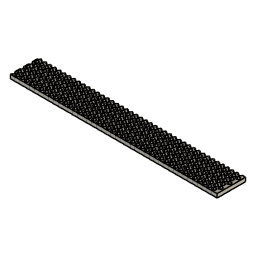
newmeshhoneycomb (Autodesk Fusion 360 design; units mm, degrees)
Autodesk Fusion 360 part; units mm, degrees
(part 1 of 3)
sketch "Sketch1" plane through (0, 0, 0) normal (0, 0, 1) x (1, 0, 0)
  line L0 (-30.9287, -0.75) -> (-29.6296, -1.5)
  line L1 (-30.9287, 0.75) -> (-30.9287, -0.75)
  line L2 (-29.6296, 1.5) -> (-30.9287, 0.75)
  line L3 (-33.3333, -1.5) -> (-32.0343, -0.75)
  line L4 (-34.6324, -0.75) -> (-33.3333, -1.5)
  line L5 (-34.6324, 0.75) -> (-34.6324, -0.75)
  line L6 (-33.3333, 1.5) -> (-34.6324, 0.75)
  line L7 (-32.0343, 0.75) -> (-33.3333, 1.5)
  line L8 (-32.0343, -0.75) -> (-32.0343, 0.75)
  line L9 (-29.225, -2.7141) -> (-29.225, -4.2141)
  line L10 (-30.3306, -2.7141) -> (-31.6296, -1.9641)
  line L11 (-31.6296, -1.9641) -> (-32.9287, -2.7141)
  line L12 (-32.9287, -2.7141) -> (-32.9287, -4.2141)
  line L13 (-32.9287, -4.2141) -> (-31.6296, -4.9641)
  line L14 (-31.6296, -4.9641) -> (-30.3306, -4.2141)
  line L15 (-30.3306, -4.2141) -> (-30.3306, -2.7141)
  line L16 (-34.0343, -2.7141) -> (-35.3333, -1.9641)
  line L17 (-35.3333, -1.9641) -> (-36.6324, -2.7141)
  line L18 (-36.6324, -2.7141) -> (-36.6324, -4.2141)
  line L19 (-36.6324, -4.2141) -> (-35.3333, -4.9641)
  line L20 (-35.3333, -4.9641) -> (-34.0343, -4.2141)
  line L21 (-34.0343, -4.2141) -> (-34.0343, -2.7141)
  line L22 (-31.0583, -5.8895) -> (-31.0583, -7.3895)
  line L23 (-39.1667, -8.6036) -> (-40.4657, -9.3536)
  line L24 (-34.762, -5.8895) -> (-34.762, -7.3895)
  line L25 (-40.4657, -9.3536) -> (-40.4657, -10.8536)
  line L26 (-29.3546, -9.3536) -> (-29.3546, -10.8536)
  line L27 (-33.463, -5.1395) -> (-34.762, -5.8895)
  line L28 (-31.0583, -7.3895) -> (-29.7593, -8.1395)
  line L29 (-30.4602, -10.8536) -> (-30.4602, -9.3536)
  line L30 (-37.8676, -10.8536) -> (-37.8676, -9.3536)
  line L31 (-32.1639, -7.3895) -> (-32.1639, -5.8895)
  line L32 (-39.1667, -11.6036) -> (-37.8676, -10.8536)
  line L33 (-36.762, -10.8536) -> (-35.463, -11.6036)
  line L34 (-35.8676, -7.3895) -> (-35.8676, -5.8895)
  line L35 (-33.0583, -10.8536) -> (-31.7593, -11.6036)
  line L36 (-35.463, -11.6036) -> (-34.1639, -10.8536)
  line L37 (-29.7593, -5.1395) -> (-31.0583, -5.8895)
  line L38 (-33.0583, -9.3536) -> (-33.0583, -10.8536)
  line L39 (-30.4602, -9.3536) -> (-31.7593, -8.6036)
  line L40 (-31.7593, -11.6036) -> (-30.4602, -10.8536)
  line L41 (-34.1639, -9.3536) -> (-35.463, -8.6036)
  line L42 (-32.1639, -5.8895) -> (-33.463, -5.1395)
  line L43 (-35.463, -8.6036) -> (-36.762, -9.3536)
  line L44 (-36.762, -9.3536) -> (-36.762, -10.8536)
  line L45 (-34.762, -7.3895) -> (-33.463, -8.1395)
  line L46 (-34.1639, -10.8536) -> (-34.1639, -9.3536)
  line L47 (-38.4657, -5.8895) -> (-38.4657, -7.3895)
  line L48 (-33.463, -8.1395) -> (-32.1639, -7.3895)
  line L49 (-31.7593, -8.6036) -> (-33.0583, -9.3536)
  line L50 (-37.8676, -9.3536) -> (-39.1667, -8.6036)
  line L51 (-35.8676, -5.8895) -> (-37.1667, -5.1395)
  line L52 (-37.1667, -8.1395) -> (-35.8676, -7.3895)
  line L53 (-37.1667, -5.1395) -> (-38.4657, -5.8895)
  line L54 (-38.4657, -7.3895) -> (-37.1667, -8.1395)
  line L55 (-40.4657, -10.8536) -> (-39.1667, -11.6036)
  line L56 (-34.8916, -12.5291) -> (-34.8916, -14.0291)
  line L57 (-43, -15.2432) -> (-44.299, -15.9932)
  line L58 (-38.5953, -12.5291) -> (-38.5953, -14.0291)
  line L59 (-44.299, -15.9932) -> (-44.299, -17.4932)
  line L60 (-33.1879, -15.9932) -> (-33.1879, -17.4932)
  line L61 (-37.2963, -11.7791) -> (-38.5953, -12.5291)
  line L62 (-34.8916, -14.0291) -> (-33.5926, -14.7791)
  line L63 (-34.2936, -17.4932) -> (-34.2936, -15.9932)
  line L64 (-33.1879, -17.4932) -> (-31.8889, -18.2432)
  line L65 (-33.5926, -14.7791) -> (-32.2936, -14.0291)
  line L66 (-30.5899, -15.9932) -> (-31.8889, -15.2432)
  line L67 (-30.5899, -17.4932) -> (-30.5899, -15.9932)
  line L68 (-29.8889, -11.7791) -> (-31.1879, -12.5291)
  line L69 (-29.4842, -15.9932) -> (-29.4842, -17.4932)
  line L70 (-31.8889, -18.2432) -> (-30.5899, -17.4932)
  line L71 (-41.701, -17.4932) -> (-41.701, -15.9932)
  line L72 (-35.9973, -14.0291) -> (-35.9973, -12.5291)
  line L73 (-43, -18.2432) -> (-41.701, -17.4932)
  line L74 (-31.8889, -15.2432) -> (-33.1879, -15.9932)
  line L75 (-40.5953, -17.4932) -> (-39.2963, -18.2432)
  line L76 (-39.701, -14.0291) -> (-39.701, -12.5291)
  line L77 (-36.8916, -17.4932) -> (-35.5926, -18.2432)
  line L78 (-39.2963, -18.2432) -> (-37.9973, -17.4932)
  line L79 (-31.1879, -14.0291) -> (-29.8889, -14.7791)
  line L80 (-33.5926, -11.7791) -> (-34.8916, -12.5291)
  line L81 (-36.8916, -15.9932) -> (-36.8916, -17.4932)
  line L82 (-34.2936, -15.9932) -> (-35.5926, -15.2432)
  line L83 (-35.5926, -18.2432) -> (-34.2936, -17.4932)
  line L84 (-37.9973, -15.9932) -> (-39.2963, -15.2432)
  line L85 (-32.2936, -12.5291) -> (-33.5926, -11.7791)
  line L86 (-35.9973, -12.5291) -> (-37.2963, -11.7791)
  line L87 (-39.2963, -15.2432) -> (-40.5953, -15.9932)
  line L88 (-40.5953, -15.9932) -> (-40.5953, -17.4932)
  line L89 (-31.1879, -12.5291) -> (-31.1879, -14.0291)
  line L90 (-38.5953, -14.0291) -> (-37.2963, -14.7791)
  line L91 (-37.9973, -17.4932) -> (-37.9973, -15.9932)
  line L92 (-32.2936, -14.0291) -> (-32.2936, -12.5291)
  line L93 (-42.299, -12.5291) -> (-42.299, -14.0291)
  line L94 (-37.2963, -14.7791) -> (-35.9973, -14.0291)
  line L95 (-35.5926, -15.2432) -> (-36.8916, -15.9932)
  line L96 (-41.701, -15.9932) -> (-43, -15.2432)
  line L97 (-39.701, -12.5291) -> (-41, -11.7791)
  line L98 (-41, -14.7791) -> (-39.701, -14.0291)
  line L99 (-41, -11.7791) -> (-42.299, -12.5291)
  line L100 (-42.299, -14.0291) -> (-41, -14.7791)
  line L101 (-44.299, -17.4932) -> (-43, -18.2432)
  line L102 (-38.725, -19.1686) -> (-38.725, -20.6686)
  line L103 (-42.4287, -19.1686) -> (-42.4287, -20.6686)
  line L104 (-41.1296, -18.4186) -> (-42.4287, -19.1686)
  line L105 (-38.725, -20.6686) -> (-37.4259, -21.4186)
  line L106 (-37.4259, -21.4186) -> (-36.1269, -20.6686)
  line L107 (-33.7222, -18.4186) -> (-35.0213, -19.1686)
  line L108 (-31.3176, -20.6686) -> (-30.0185, -21.4186)
  line L109 (-33.7222, -21.4186) -> (-32.4232, -20.6686)
  line L110 (-39.8306, -20.6686) -> (-39.8306, -19.1686)
  line L111 (-32.4232, -20.6686) -> (-32.4232, -19.1686)
  line L112 (-32.4232, -19.1686) -> (-33.7222, -18.4186)
  line L113 (-43.5343, -20.6686) -> (-43.5343, -19.1686)
  line L114 (-35.0213, -20.6686) -> (-33.7222, -21.4186)
  line L115 (-37.4259, -18.4186) -> (-38.725, -19.1686)
  line L116 (-30.0185, -18.4186) -> (-31.3176, -19.1686)
  line L117 (-36.1269, -19.1686) -> (-37.4259, -18.4186)
  line L118 (-39.8306, -19.1686) -> (-41.1296, -18.4186)
  line L119 (-31.3176, -19.1686) -> (-31.3176, -20.6686)
  line L120 (-35.0213, -19.1686) -> (-35.0213, -20.6686)
  line L121 (-42.4287, -20.6686) -> (-41.1296, -21.4186)
  line L122 (-36.1269, -20.6686) -> (-36.1269, -19.1686)
  line L123 (-46.1324, -19.1686) -> (-46.1324, -20.6686)
  line L124 (-41.1296, -21.4186) -> (-39.8306, -20.6686)
  line L125 (-43.5343, -19.1686) -> (-44.8333, -18.4186)
  line L126 (-44.8333, -21.4186) -> (-43.5343, -20.6686)
  line L127 (-44.8333, -18.4186) -> (-46.1324, -19.1686)
  line L128 (-46.1324, -20.6686) -> (-44.8333, -21.4186)
  line L129 (-101.9101, -19.1686) -> (-101.9101, -20.6686)
  line L130 (-99.3121, -19.1686) -> (-100.6111, -18.4186)
  line L131 (-95.5343, -19.1686) -> (-96.8333, -18.4186)
  line L132 (-98.1324, -19.1686) -> (-98.1324, -20.6686)
  line L133 (-95.5343, -20.6686) -> (-95.5343, -19.1686)
  line L134 (-96.8333, -18.4186) -> (-98.1324, -19.1686)
  line L135 (-100.6111, -21.4186) -> (-99.3121, -20.6686)
  line L136 (-103.0158, -19.1686) -> (-104.3148, -18.4186)
  line L137 (-106.7195, -19.1686) -> (-108.0185, -18.4186)
  line L138 (-109.3176, -20.6686) -> (-108.0185, -21.4186)
  line L139 (-110.4232, -19.1686) -> (-111.7222, -18.4186)
  line L140 (-103.7805, -15.9932) -> (-103.7805, -17.4932)
  line L141 (-102.8861, -12.5291) -> (-104.1852, -11.7791)
  line L142 (-106.5899, -14.0291) -> (-106.5899, -12.5291)
  line L143 (-108.5899, -15.9932) -> (-109.8889, -15.2432)
  line L144 (-105.4842, -14.0291) -> (-104.1852, -14.7791)
  line L145 (-106.1852, -15.2432) -> (-107.4842, -15.9932)
  line L146 (-109.1879, -12.5291) -> (-109.1879, -14.0291)
  line L147 (-105.4842, -12.5291) -> (-105.4842, -14.0291)
  line L148 (-107.4842, -17.4932) -> (-106.1852, -18.2432)
  line L149 (-107.8889, -11.7791) -> (-109.1879, -12.5291)
  line L150 (-109.8889, -15.2432) -> (-111.1879, -15.9932)
  line L151 (-88.1269, -20.6686) -> (-88.1269, -19.1686)
  line L152 (-91.8306, -19.1686) -> (-93.1296, -18.4186)
  line L153 (-93.1296, -21.4186) -> (-91.8306, -20.6686)
  line L154 (-90.725, -20.6686) -> (-89.4259, -21.4186)
  line L155 (-94.4287, -19.1686) -> (-94.4287, -20.6686)
  line L156 (-94.4287, -20.6686) -> (-93.1296, -21.4186)
  line L157 (-89.4259, -21.4186) -> (-88.1269, -20.6686)
  line L158 (-90.725, -19.1686) -> (-90.725, -20.6686)
  line L159 (-93.1296, -18.4186) -> (-94.4287, -19.1686)
  line L160 (-89.4259, -18.4186) -> (-90.725, -19.1686)
  line L161 (-101.9101, -20.6686) -> (-100.6111, -21.4186)
  line L162 (-96.8333, -21.4186) -> (-95.5343, -20.6686)
  line L163 (-99.3121, -20.6686) -> (-99.3121, -19.1686)
  line L164 (-95.4787, -14.0291) -> (-95.4787, -12.5291)
  line L165 (-96.7778, -11.7791) -> (-98.0768, -12.5291)
  line L166 (-97.4787, -15.9932) -> (-98.7778, -15.2432)
  line L167 (-101.1824, -15.9932) -> (-102.4815, -15.2432)
  line L168 (-98.7778, -15.2432) -> (-100.0768, -15.9932)
  line L169 (-96.7778, -14.7791) -> (-95.4787, -14.0291)
  line L170 (-101.1824, -17.4932) -> (-101.1824, -15.9932)
  line L171 (-95.4787, -12.5291) -> (-96.7778, -11.7791)
  line L172 (-101.7805, -12.5291) -> (-101.7805, -14.0291)
  line L173 (-98.7778, -18.2432) -> (-97.4787, -17.4932)
  line L174 (-111.3333, 1.5) -> (-112.6324, 0.75)
  line L175 (-99.1824, -12.5291) -> (-100.4815, -11.7791)
  line L176 (-100.4815, -14.7791) -> (-99.1824, -14.0291)
  line L177 (-111.463, -8.1395) -> (-110.1639, -7.3895)
  line L178 (-98.0768, -12.5291) -> (-98.0768, -14.0291)
  line L179 (-104.1852, -14.7791) -> (-102.8861, -14.0291)
  line L180 (-107.4842, -15.9932) -> (-107.4842, -17.4932)
  line L181 (-104.8861, -17.4932) -> (-104.8861, -15.9932)
  line L182 (-106.1852, -18.2432) -> (-104.8861, -17.4932)
  line L183 (-104.1852, -11.7791) -> (-105.4842, -12.5291)
  line L184 (-111.1879, -15.9932) -> (-111.1879, -17.4932)
  line L185 (-111.1879, -17.4932) -> (-109.8889, -18.2432)
  line L186 (-100.6111, -18.4186) -> (-101.9101, -19.1686)
  line L187 (-98.1324, -20.6686) -> (-96.8333, -21.4186)
  line L188 (-90.5953, -12.5291) -> (-90.5953, -14.0291)
  line L189 (-91.701, -14.0291) -> (-91.701, -12.5291)
  line L190 (-88.8916, -15.9932) -> (-88.8916, -17.4932)
  line L191 (-91.2963, -18.2432) -> (-89.9973, -17.4932)
  line L192 (-93, -11.7791) -> (-94.299, -12.5291)
  line L193 (-89.9973, -15.9932) -> (-91.2963, -15.2432)
  line L194 (-91.701, -12.5291) -> (-93, -11.7791)
  line L195 (-92.5953, -15.9932) -> (-92.5953, -17.4932)
  line L196 (-91.2963, -15.2432) -> (-92.5953, -15.9932)
  line L197 (-94.299, -12.5291) -> (-94.299, -14.0291)
  line L198 (-111.5926, -14.7791) -> (-110.2936, -14.0291)
  line L199 (-89.2963, -11.7791) -> (-90.5953, -12.5291)
  line L200 (-92.5953, -17.4932) -> (-91.2963, -18.2432)
  line L201 (-95, -18.2432) -> (-93.701, -17.4932)
  line L202 (-93.701, -17.4932) -> (-93.701, -15.9932)
  line L203 (-112.6324, -0.75) -> (-111.3333, -1.5)
  line L204 (-111.7222, -21.4186) -> (-110.4232, -20.6686)
  line L205 (-103.0158, -20.6686) -> (-103.0158, -19.1686)
  line L206 (-104.3148, -18.4186) -> (-105.6139, -19.1686)
  line L207 (-105.6139, -20.6686) -> (-104.3148, -21.4186)
  line L208 (-109.3176, -19.1686) -> (-109.3176, -20.6686)
  line L209 (-91.8306, -20.6686) -> (-91.8306, -19.1686)
  line L210 (-88.1269, -19.1686) -> (-89.4259, -18.4186)
  line L211 (-94.299, -14.0291) -> (-93, -14.7791)
  line L212 (-89.9973, -17.4932) -> (-89.9973, -15.9932)
  line L213 (-87.9973, -12.5291) -> (-89.2963, -11.7791)
  line L214 (-93, -14.7791) -> (-91.701, -14.0291)
  line L215 (-58.1639, -7.3895) -> (-58.1639, -5.8895)
  line L216 (-89.8121, -4.2141) -> (-89.8121, -2.7141)
  line L217 (-66.4657, -9.3536) -> (-66.4657, -10.8536)
  line L218 (-57.6296, -1.9641) -> (-58.9287, -2.7141)
  line L219 (-63.1111, -1.5) -> (-61.8121, -0.75)
  line L220 (-93.5158, -2.7141) -> (-94.8148, -1.9641)
  line L221 (-71.2195, -4.2141) -> (-71.2195, -2.7141)
  line L222 (-73.0528, -5.8895) -> (-74.3519, -5.1395)
  line L223 (-103.9259, -1.5) -> (-102.6269, -0.75)
  line L224 (-52.0556, -8.1395) -> (-50.7565, -7.3895)
  line L225 (-63.8121, -4.2141) -> (-63.8121, -2.7141)
  line L226 (-56.9287, -0.75) -> (-55.6296, -1.5)
  line L227 (-91.1111, -1.9641) -> (-92.4101, -2.7141)
  line L228 (-45.3491, -10.8536) -> (-45.3491, -9.3536)
  line L229 (-58.9287, -4.2141) -> (-57.6296, -4.9641)
  line L230 (-105.225, -0.75) -> (-103.9259, -1.5)
  line L231 (-73.8176, -4.2141) -> (-72.5185, -4.9641)
  line L232 (-90.4657, -5.8895) -> (-90.4657, -7.3895)
  line L233 (-68.8148, -4.9641) -> (-67.5158, -4.2141)
  line L234 (-75.6509, -7.3895) -> (-74.3519, -8.1395)
  line L235 (-52.0556, -5.1395) -> (-53.3546, -5.8895)
  line L236 (-92.8148, -1.5) -> (-91.5158, -0.75)
  line L237 (-42.8148, -1.9641) -> (-44.1139, -2.7141)
  line L238 (-92.4657, -9.3536) -> (-92.4657, -10.8536)
  line L239 (-74.9232, -4.2141) -> (-74.9232, -2.7141)
  line L240 (-63.8676, -9.3536) -> (-65.1667, -8.6036)
  line L241 (-71.2195, -2.7141) -> (-72.5185, -1.9641)
  line L242 (-73.9472, -9.3536) -> (-73.9472, -10.8536)
  line L243 (-53.9259, -1.9641) -> (-55.225, -2.7141)
  line L244 (-54.4602, -5.8895) -> (-55.7593, -5.1395)
  line L245 (-94.2435, -7.3895) -> (-92.9444, -8.1395)
  line L246 (-74.3519, -8.1395) -> (-73.0528, -7.3895)
  line L247 (-70.1139, -2.7141) -> (-70.1139, -4.2141)
  line L248 (-44.2435, -9.3536) -> (-44.2435, -10.8536)
  line L249 (-75.5213, -0.75) -> (-74.2222, -1.5)
  line L250 (-90.4101, -0.75) -> (-89.1111, -1.5)
  line L251 (-103.5213, -4.2141) -> (-102.2222, -4.9641)
  line L252 (-76.2222, -4.9641) -> (-74.9232, -4.2141)
  line L253 (-68.9444, -8.6036) -> (-70.2435, -9.3536)
  line L254 (-104.6269, -4.2141) -> (-104.6269, -2.7141)
  line L255 (-103.5213, -2.7141) -> (-103.5213, -4.2141)
  line L256 (-71.3491, -9.3536) -> (-72.6481, -8.6036)
  line L257 (-74.3519, -5.1395) -> (-75.6509, -5.8895)
  line L258 (-59.3333, -1.5) -> (-58.0343, -0.75)
  line L259 (-93.5158, -4.2141) -> (-93.5158, -2.7141)
  line L260 (-77.5213, -4.2141) -> (-76.2222, -4.9641)
  line L261 (-41.6454, -9.3536) -> (-42.9444, -8.6036)
  line L262 (-65.1111, -4.9641) -> (-63.8121, -4.2141)
  line L263 (-89.8676, -10.8536) -> (-89.8676, -9.3536)
  line L264 (-55.225, -4.2141) -> (-53.9259, -4.9641)
  line L265 (-56.4602, -10.8536) -> (-56.4602, -9.3536)
  line L266 (-74.2222, -1.5) -> (-72.9232, -0.75)
  line L267 (-41.5158, -2.7141) -> (-42.8148, -1.9641)
  line L268 (-73.8176, -2.7141) -> (-73.8176, -4.2141)
  line L269 (-76.2222, -1.9641) -> (-77.5213, -2.7141)
  line L270 (-63.8121, -2.7141) -> (-65.1111, -1.9641)
  line L271 (-47.9472, -9.3536) -> (-47.9472, -10.8536)
  line L272 (-91.1111, -4.9641) -> (-89.8121, -4.2141)
  line L273 (-65.1111, -1.9641) -> (-66.4101, -2.7141)
  line L274 (-54.0556, -8.6036) -> (-55.3546, -9.3536)
  line L275 (-73.0528, -7.3895) -> (-73.0528, -5.8895)
  line L276 (-50.7565, -7.3895) -> (-50.7565, -5.8895)
  line L277 (-94.1139, -0.75) -> (-92.8148, -1.5)
  line L278 (-70.6481, -8.1395) -> (-69.3491, -7.3895)
  line L279 (-49.9101, -20.6686) -> (-48.6111, -21.4186)
  line L280 (-82.9287, -0.75) -> (-81.6296, -1.5)
  line L281 (-78.3148, -21.4186) -> (-77.0158, -20.6686)
  line L282 (-63.9973, -15.9932) -> (-65.2963, -15.2432)
  line L283 (-88.8916, -17.4932) -> (-87.5926, -18.2432)
  line L284 (-49.7805, -14.0291) -> (-48.4815, -14.7791)
  line L285 (-83.8889, -15.2432) -> (-85.1879, -15.9932)
  line L286 (-45.4787, -17.4932) -> (-45.4787, -15.9932)
  line L287 (-60.762, -7.3895) -> (-59.463, -8.1395)
  line L288 (-110.1639, -7.3895) -> (-110.1639, -5.8895)
  line L289 (-83.6296, -4.9641) -> (-82.3306, -4.2141)
  line L290 (-51.0158, -19.1686) -> (-52.3148, -18.4186)
  line L291 (-109.7593, -8.6036) -> (-111.0583, -9.3536)
  line L292 (-48.6111, -18.4186) -> (-49.9101, -19.1686)
  line L293 (-107.3546, -9.3536) -> (-107.3546, -10.8536)
  line L294 (-109.0583, -5.8895) -> (-109.0583, -7.3895)
  line L295 (-78.8861, -17.4932) -> (-78.8861, -15.9932)
  line L296 (-70.299, -17.4932) -> (-69, -18.2432)
  line L297 (-50.4815, -15.2432) -> (-51.7805, -15.9932)
  line L298 (-82.3306, -2.7141) -> (-83.6296, -1.9641)
  line L299 (-61.9973, -12.5291) -> (-63.2963, -11.7791)
  line L300 (-81.7593, -5.1395) -> (-83.0583, -5.8895)
  line L301 (-60.2936, -17.4932) -> (-60.2936, -15.9932)
  line L302 (-101.5213, -0.75) -> (-100.2222, -1.5)
  line L303 (-60.6324, -0.75) -> (-59.3333, -1.5)
  line L304 (-107.7593, -8.1395) -> (-106.4602, -7.3895)
  line L305 (-53.6139, -19.1686) -> (-53.6139, -20.6686)
  line L306 (-50.4815, -18.2432) -> (-49.1824, -17.4932)
  line L307 (-78.1852, -14.7791) -> (-76.8861, -14.0291)
  line L308 (-82.4602, -10.8536) -> (-82.4602, -9.3536)
  line L309 (-85.0583, -9.3536) -> (-85.0583, -10.8536)
  line L310 (-108.4602, -9.3536) -> (-109.7593, -8.6036)
  line L311 (-77.7805, -17.4932) -> (-76.4815, -18.2432)
  line L312 (-79.6139, -20.6686) -> (-78.3148, -21.4186)
  line L313 (-61.0213, -20.6686) -> (-59.7222, -21.4186)
  line L314 (-108.4602, -10.8536) -> (-108.4602, -9.3536)
  line L315 (-46.0768, -12.5291) -> (-46.0768, -14.0291)
  line L316 (-84.2936, -12.5291) -> (-85.5926, -11.7791)
  line L317 (-64.725, -19.1686) -> (-64.725, -20.6686)
  line L318 (-69.5343, -20.6686) -> (-69.5343, -19.1686)
  line L319 (-52.3148, -18.4186) -> (-53.6139, -19.1686)
  line L320 (-111.0583, -9.3536) -> (-111.0583, -10.8536)
  line L321 (-83.0583, -7.3895) -> (-81.7593, -8.1395)
  line L322 (-76.8861, -12.5291) -> (-78.1852, -11.7791)
  line L323 (-52.1852, -11.7791) -> (-53.4842, -12.5291)
  line L324 (-49.9101, -19.1686) -> (-49.9101, -20.6686)
  line L325 (-48.4815, -11.7791) -> (-49.7805, -12.5291)
  line L326 (-76.4815, -18.2432) -> (-75.1824, -17.4932)
  line L327 (-84.9287, -2.7141) -> (-84.9287, -4.2141)
  line L328 (-59.7222, -18.4186) -> (-61.0213, -19.1686)
  line L329 (-109.0583, -7.3895) -> (-107.7593, -8.1395)
  line L330 (-86.6324, -0.75) -> (-85.3333, -1.5)
  line L331 (-50.8861, -14.0291) -> (-50.8861, -12.5291)
  line L332 (-106.4602, -7.3895) -> (-106.4602, -5.8895)
  line L333 (-71.4787, -17.4932) -> (-71.4787, -15.9932)
  line L334 (-72.0768, -14.0291) -> (-70.7778, -14.7791)
  line L335 (-76.8861, -14.0291) -> (-76.8861, -12.5291)
  line L336 (-64.725, -20.6686) -> (-63.4259, -21.4186)
  line L337 (-86.2936, -17.4932) -> (-86.2936, -15.9932)
  line L338 (-78.7565, -9.3536) -> (-80.0556, -8.6036)
  line L339 (-46.0768, -14.0291) -> (-44.7778, -14.7791)
  line L340 (-88.762, -9.3536) -> (-88.762, -10.8536)
  line L341 (-52.1852, -14.7791) -> (-50.8861, -14.0291)
  line L342 (-71.4787, -15.9932) -> (-72.7778, -15.2432)
  line L343 (-73.3121, -20.6686) -> (-73.3121, -19.1686)
  line L344 (-79.3546, -5.8895) -> (-79.3546, -7.3895)
  line L345 (-53.6139, -20.6686) -> (-52.3148, -21.4186)
  line L346 (-70.8333, -21.4186) -> (-69.5343, -20.6686)
  line L347 (-75.7805, -14.0291) -> (-74.4815, -14.7791)
  line L348 (-81.4842, -17.4932) -> (-80.1852, -18.2432)
  line L349 (-101.0528, -10.8536) -> (-101.0528, -9.3536)
  line L350 (-85.5926, -11.7791) -> (-86.8916, -12.5291)
  line L351 (-80.4602, -7.3895) -> (-80.4602, -5.8895)
  line L352 (-43.4787, -14.0291) -> (-43.4787, -12.5291)
  line L353 (-70.299, -15.9932) -> (-70.299, -17.4932)
  line L354 (-79.4842, -12.5291) -> (-79.4842, -14.0291)
  line L355 (-86.1639, -10.8536) -> (-86.1639, -9.3536)
  line L356 (-47.1824, -14.0291) -> (-47.1824, -12.5291)
  line L357 (-58.2936, -12.5291) -> (-59.5926, -11.7791)
  line L358 (-100.3519, -8.1395) -> (-99.0528, -7.3895)
  line L359 (-85.463, -8.1395) -> (-84.1639, -7.3895)
  line L360 (-69.5343, -19.1686) -> (-70.8333, -18.4186)
  line L361 (-84.1639, -5.8895) -> (-85.463, -5.1395)
  line L362 (-58.4232, -19.1686) -> (-59.7222, -18.4186)
  line L363 (-82.5899, -15.9932) -> (-83.8889, -15.2432)
  line L364 (-52.3148, -21.4186) -> (-51.0158, -20.6686)
  line L365 (-65.8306, -19.1686) -> (-67.1296, -18.4186)
  line L366 (-84.1639, -7.3895) -> (-84.1639, -5.8895)
  line L367 (-79.9259, -1.9641) -> (-81.225, -2.7141)
  line L368 (-63.4259, -21.4186) -> (-62.1269, -20.6686)
  line L369 (-72.7778, -15.2432) -> (-74.0768, -15.9932)
  line L370 (-46.7778, -15.2432) -> (-48.0768, -15.9932)
  line L371 (-56.0185, -21.4186) -> (-54.7195, -20.6686)
  line L372 (-81.4842, -15.9932) -> (-81.4842, -17.4932)
  line L373 (-77.5213, -2.7141) -> (-77.5213, -4.2141)
  line L374 (-46.7778, -18.2432) -> (-45.4787, -17.4932)
  line L375 (-81.7593, -8.1395) -> (-80.4602, -7.3895)
  line L376 (-54.1852, -18.2432) -> (-52.8861, -17.4932)
  line L377 (-65.2963, -15.2432) -> (-66.5953, -15.9932)
  line L378 (-62.8916, -15.9932) -> (-62.8916, -17.4932)
  line L379 (-52.8861, -15.9932) -> (-54.1852, -15.2432)
  line L380 (-83.6296, -1.9641) -> (-84.9287, -2.7141)
  line L381 (-69.4787, -14.0291) -> (-69.4787, -12.5291)
  line L382 (-51.7805, -15.9932) -> (-51.7805, -17.4932)
  line L383 (-65.8306, -20.6686) -> (-65.8306, -19.1686)
  line L384 (-76.3519, -8.6036) -> (-77.6509, -9.3536)
  line L385 (-57.8889, -18.2432) -> (-56.5899, -17.4932)
  line L386 (-82.3306, -4.2141) -> (-82.3306, -2.7141)
  line L387 (-102.7565, -7.3895) -> (-102.7565, -5.8895)
  line L388 (-75.1824, -15.9932) -> (-76.4815, -15.2432)
  line L389 (-88.6324, -4.2141) -> (-87.3333, -4.9641)
  line L390 (-51.7805, -17.4932) -> (-50.4815, -18.2432)
  line L391 (-65.2963, -18.2432) -> (-63.9973, -17.4932)
  line L392 (-52.8861, -17.4932) -> (-52.8861, -15.9932)
  line L393 (-44.7778, -11.7791) -> (-46.0768, -12.5291)
  line L394 (-63.4259, -18.4186) -> (-64.725, -19.1686)
  line L395 (-76.7565, -7.3895) -> (-76.7565, -5.8895)
  line L396 (-55.8889, -14.7791) -> (-54.5899, -14.0291)
  line L397 (-70.7778, -14.7791) -> (-69.4787, -14.0291)
  line L398 (-65.701, -14.0291) -> (-65.701, -12.5291)
  line L399 (-74.4815, -14.7791) -> (-73.1824, -14.0291)
  line L400 (-105.3546, -7.3895) -> (-104.0556, -8.1395)
  line L401 (-59.1879, -15.9932) -> (-59.1879, -17.4932)
  line L402 (-49.7805, -12.5291) -> (-49.7805, -14.0291)
  line L403 (-83.7593, -8.6036) -> (-85.0583, -9.3536)
  line L404 (-48.0768, -17.4932) -> (-46.7778, -18.2432)
  line L405 (-49.1824, -17.4932) -> (-49.1824, -15.9932)
  line L406 (-80.0556, -8.6036) -> (-81.3546, -9.3536)
  line L407 (-48.6111, -21.4186) -> (-47.3121, -20.6686)
  line L408 (-102.3519, -8.6036) -> (-103.6509, -9.3536)
  line L409 (-86.762, -5.8895) -> (-86.762, -7.3895)
  line L410 (-48.4815, -14.7791) -> (-47.1824, -14.0291)
  line L411 (-81.6296, -1.5) -> (-80.3306, -0.75)
  line L412 (-73.1824, -12.5291) -> (-74.4815, -11.7791)
  line L413 (-85.463, -5.1395) -> (-86.762, -5.8895)
  line L414 (-79.3546, -7.3895) -> (-78.0556, -8.1395)
  line L415 (-105.3546, -5.8895) -> (-105.3546, -7.3895)
  line L416 (-61.5926, -18.2432) -> (-60.2936, -17.4932)
  line L417 (-104.0556, -8.1395) -> (-102.7565, -7.3895)
  line L418 (-67.701, -15.9932) -> (-69, -15.2432)
  line L419 (-87.3333, -1.9641) -> (-88.6324, -2.7141)
  line L420 (-85.5926, -14.7791) -> (-84.2936, -14.0291)
  line L421 (-85.1879, -17.4932) -> (-83.8889, -18.2432)
  line L422 (-50.8861, -12.5291) -> (-52.1852, -11.7791)
  line L423 (-86.8916, -12.5291) -> (-86.8916, -14.0291)
  line L424 (-79.225, -0.75) -> (-77.9259, -1.5)
  line L425 (-56.5899, -15.9932) -> (-57.8889, -15.2432)
  line L426 (-72.7778, -18.2432) -> (-71.4787, -17.4932)
  line L427 (-56.0185, -18.4186) -> (-57.3176, -19.1686)
  line L428 (-87.463, -8.6036) -> (-88.762, -9.3536)
  line L429 (-78.0556, -5.1395) -> (-79.3546, -5.8895)
  line L430 (-101.6509, -7.3895) -> (-100.3519, -8.1395)
  line L431 (-79.9259, -4.9641) -> (-78.6269, -4.2141)
  line L432 (-73.3121, -19.1686) -> (-74.6111, -18.4186)
  line L433 (-83.1879, -12.5291) -> (-83.1879, -14.0291)
  line L434 (-104.7565, -9.3536) -> (-106.0556, -8.6036)
  line L435 (-83.8889, -18.2432) -> (-82.5899, -17.4932)
  line L436 (-63.2963, -14.7791) -> (-61.9973, -14.0291)
  line L437 (-69.4787, -12.5291) -> (-70.7778, -11.7791)
  line L438 (-87.8676, -7.3895) -> (-87.8676, -5.8895)
  line L439 (-57.3176, -19.1686) -> (-57.3176, -20.6686)
  line L440 (-82.5899, -17.4932) -> (-82.5899, -15.9932)
  line L441 (-45.4787, -15.9932) -> (-46.7778, -15.2432)
  line L442 (-56.5899, -17.4932) -> (-56.5899, -15.9932)
  line L443 (-87.5926, -18.2432) -> (-86.2936, -17.4932)
  line L444 (-48.0768, -15.9932) -> (-48.0768, -17.4932)
  line L445 (-75.9101, -20.6686) -> (-74.6111, -21.4186)
  line L446 (-82.4602, -9.3536) -> (-83.7593, -8.6036)
  line L447 (-80.4602, -5.8895) -> (-81.7593, -5.1395)
  line L448 (-98.5185, -4.9641) -> (-97.2195, -4.2141)
  line L449 (-101.6509, -5.8895) -> (-101.6509, -7.3895)
  line L450 (-95.3491, -5.8895) -> (-96.6481, -5.1395)
  line L451 (-106.0556, -8.6036) -> (-107.3546, -9.3536)
  line L452 (-44.7778, -14.7791) -> (-43.4787, -14.0291)
  line L453 (-76.4815, -15.2432) -> (-77.7805, -15.9932)
  line L454 (-86.8916, -14.0291) -> (-85.5926, -14.7791)
  line L455 (-101.0528, -9.3536) -> (-102.3519, -8.6036)
  line L456 (-80.5899, -14.0291) -> (-80.5899, -12.5291)
  line L457 (-73.1824, -14.0291) -> (-73.1824, -12.5291)
  line L458 (-78.0556, -8.1395) -> (-76.7565, -7.3895)
  line L459 (-103.6509, -9.3536) -> (-103.6509, -10.8536)
  line L460 (-54.7195, -19.1686) -> (-56.0185, -18.4186)
  line L461 (-85.3333, -1.5) -> (-84.0343, -0.75)
  line L462 (-58.2936, -14.0291) -> (-58.2936, -12.5291)
  line L463 (-57.1879, -12.5291) -> (-57.1879, -14.0291)
  line L464 (-57.8889, -15.2432) -> (-59.1879, -15.9932)
  line L465 (-77.6509, -9.3536) -> (-77.6509, -10.8536)
  line L466 (-60.8916, -14.0291) -> (-59.5926, -14.7791)
  line L467 (-67.1296, -18.4186) -> (-68.4287, -19.1686)
  line L468 (-43.4787, -12.5291) -> (-44.7778, -11.7791)
  line L469 (-51.0158, -20.6686) -> (-51.0158, -19.1686)
  line L470 (-86.0343, -4.2141) -> (-86.0343, -2.7141)
  line L471 (-47.1824, -12.5291) -> (-48.4815, -11.7791)
  line L472 (-47.3121, -20.6686) -> (-47.3121, -19.1686)
  line L473 (-53.4842, -12.5291) -> (-53.4842, -14.0291)
  line L474 (-83.0583, -5.8895) -> (-83.0583, -7.3895)
  line L475 (-53.4842, -14.0291) -> (-52.1852, -14.7791)
  line L476 (-60.2936, -15.9932) -> (-61.5926, -15.2432)
  line L477 (-67.701, -17.4932) -> (-67.701, -15.9932)
  line L478 (-79.4842, -14.0291) -> (-78.1852, -14.7791)
  line L479 (-68.4287, -20.6686) -> (-67.1296, -21.4186)
  line L480 (-49.1824, -15.9932) -> (-50.4815, -15.2432)
  line L481 (-86.0343, -2.7141) -> (-87.3333, -1.9641)
  line L482 (-87.3333, -4.9641) -> (-86.0343, -4.2141)
  line L483 (-81.8889, -14.7791) -> (-80.5899, -14.0291)
  line L484 (-81.3546, -9.3536) -> (-81.3546, -10.8536)
  line L485 (-47.3121, -19.1686) -> (-48.6111, -18.4186)
  line L486 (-69, -18.2432) -> (-67.701, -17.4932)
  line L487 (-104.7565, -10.8536) -> (-104.7565, -9.3536)
  line L488 (-86.1639, -9.3536) -> (-87.463, -8.6036)
  line L489 (-99.8176, -2.7141) -> (-99.8176, -4.2141)
  line L490 (-81.225, -4.2141) -> (-79.9259, -4.9641)
  line L491 (-83.1879, -14.0291) -> (-81.8889, -14.7791)
  line L492 (-66.5953, -17.4932) -> (-65.2963, -18.2432)
  line L493 (-72.0768, -12.5291) -> (-72.0768, -14.0291)
  line L494 (-81.225, -2.7141) -> (-81.225, -4.2141)
  line L495 (-96.1139, -2.7141) -> (-96.1139, -4.2141)
  line L496 (-59.7222, -21.4186) -> (-58.4232, -20.6686)
  line L497 (-85.1879, -15.9932) -> (-85.1879, -17.4932)
  line L498 (-61.5926, -15.2432) -> (-62.8916, -15.9932)
  line L499 (-74.4815, -11.7791) -> (-75.7805, -12.5291)
  line L500 (-94.8148, -1.9641) -> (-96.1139, -2.7141)
  line L501 (-86.762, -7.3895) -> (-85.463, -8.1395)
  line L502 (-99.0528, -7.3895) -> (-99.0528, -5.8895)
  line L503 (-70.7778, -11.7791) -> (-72.0768, -12.5291)
  line L504 (-59.5926, -11.7791) -> (-60.8916, -12.5291)
  line L505 (-74.0768, -17.4932) -> (-72.7778, -18.2432)
  line L506 (-78.6269, -2.7141) -> (-79.9259, -1.9641)
  line L507 (-106.4602, -5.8895) -> (-107.7593, -5.1395)
  line L508 (-84.2936, -14.0291) -> (-84.2936, -12.5291)
  line L509 (-100.2222, -1.5) -> (-98.9232, -0.75)
  line L510 (-80.1852, -18.2432) -> (-78.8861, -17.4932)
  line L511 (-99.8176, -4.2141) -> (-98.5185, -4.9641)
  line L512 (-75.7805, -12.5291) -> (-75.7805, -14.0291)
  line L513 (-78.6269, -4.2141) -> (-78.6269, -2.7141)
  line L514 (-109.6296, -1.9641) -> (-110.9287, -2.7141)
  line L515 (-86.2936, -15.9932) -> (-87.5926, -15.2432)
  line L516 (-78.7565, -10.8536) -> (-78.7565, -9.3536)
  line L517 (-67.1296, -21.4186) -> (-65.8306, -20.6686)
  line L518 (-75.1824, -17.4932) -> (-75.1824, -15.9932)
  line L519 (-81.8889, -11.7791) -> (-83.1879, -12.5291)
  line L520 (-64.5953, -14.0291) -> (-63.2963, -14.7791)
  line L521 (-72.1324, -19.1686) -> (-72.1324, -20.6686)
  line L522 (-69, -15.2432) -> (-70.299, -15.9932)
  line L523 (-54.5899, -14.0291) -> (-54.5899, -12.5291)
  line L524 (-88.6324, -2.7141) -> (-88.6324, -4.2141)
  line L525 (-74.0768, -15.9932) -> (-74.0768, -17.4932)
  line L526 (-108.3306, -4.2141) -> (-108.3306, -2.7141)
  line L527 (-57.3176, -20.6686) -> (-56.0185, -21.4186)
  line L528 (-76.7565, -5.8895) -> (-78.0556, -5.1395)
  line L529 (-77.7805, -15.9932) -> (-77.7805, -17.4932)
  line L530 (-59.5926, -14.7791) -> (-58.2936, -14.0291)
  line L531 (-67, -14.7791) -> (-65.701, -14.0291)
  line L532 (-97.2195, -2.7141) -> (-98.5185, -1.9641)
  line L533 (-68.299, -12.5291) -> (-68.299, -14.0291)
  line L534 (-80.1852, -15.2432) -> (-81.4842, -15.9932)
  line L535 (-68.299, -14.0291) -> (-67, -14.7791)
  line L536 (-80.5899, -12.5291) -> (-81.8889, -11.7791)
  line L537 (-77.9259, -1.5) -> (-76.6269, -0.75)
  line L538 (-96.5185, -1.5) -> (-95.2195, -0.75)
  line L539 (-74.6111, -21.4186) -> (-73.3121, -20.6686)
  line L540 (-84.9287, -4.2141) -> (-83.6296, -4.9641)
  line L541 (-55.4842, -17.4932) -> (-54.1852, -18.2432)
  line L542 (-57.1879, -14.0291) -> (-55.8889, -14.7791)
  line L543 (-97.2195, -4.2141) -> (-97.2195, -2.7141)
  line L544 (-62.1269, -19.1686) -> (-63.4259, -18.4186)
  line L545 (-63.9973, -17.4932) -> (-63.9973, -15.9932)
  line L546 (-67, -11.7791) -> (-68.299, -12.5291)
  line L547 (-61.9973, -14.0291) -> (-61.9973, -12.5291)
  line L548 (-75.9101, -19.1686) -> (-75.9101, -20.6686)
  line L549 (-61.0213, -19.1686) -> (-61.0213, -20.6686)
  line L550 (-96.2435, -9.3536) -> (-96.2435, -10.8536)
  line L551 (-78.1852, -11.7791) -> (-79.4842, -12.5291)
  line L552 (-58.4232, -20.6686) -> (-58.4232, -19.1686)
  line L553 (-74.6111, -18.4186) -> (-75.9101, -19.1686)
  line L554 (-104.0556, -5.1395) -> (-105.3546, -5.8895)
  line L555 (-68.4287, -19.1686) -> (-68.4287, -20.6686)
  line L556 (-105.9259, -1.9641) -> (-107.225, -2.7141)
  line L557 (-96.1139, -4.2141) -> (-94.8148, -4.9641)
  line L558 (-59.463, -5.1395) -> (-60.762, -5.8895)
  line L559 (-100.3519, -5.1395) -> (-101.6509, -5.8895)
  line L560 (-62.8916, -17.4932) -> (-61.5926, -18.2432)
  line L561 (-64.5953, -12.5291) -> (-64.5953, -14.0291)
  line L562 (-100.9232, -4.2141) -> (-100.9232, -2.7141)
  line L563 (-99.9472, -9.3536) -> (-99.9472, -10.8536)
  line L564 (-102.2222, -4.9641) -> (-100.9232, -4.2141)
  line L565 (-96.6481, -8.1395) -> (-95.3491, -7.3895)
  line L566 (-44.1139, -4.2141) -> (-42.8148, -4.9641)
  line L567 (-97.3491, -9.3536) -> (-98.6481, -8.6036)
  line L568 (-54.7195, -20.6686) -> (-54.7195, -19.1686)
  line L569 (-78.8861, -15.9932) -> (-80.1852, -15.2432)
  line L570 (-60.8916, -12.5291) -> (-60.8916, -14.0291)
  line L571 (-70.8333, -18.4186) -> (-72.1324, -19.1686)
  line L572 (-54.5899, -12.5291) -> (-55.8889, -11.7791)
  line L573 (-66.5953, -15.9932) -> (-66.5953, -17.4932)
  line L574 (-102.7565, -5.8895) -> (-104.0556, -5.1395)
  line L575 (-104.6269, -2.7141) -> (-105.9259, -1.9641)
  line L576 (-105.9259, -4.9641) -> (-104.6269, -4.2141)
  line L577 (-95.3491, -7.3895) -> (-95.3491, -5.8895)
  line L578 (-110.9287, -2.7141) -> (-110.9287, -4.2141)
  line L579 (-110.9287, -4.2141) -> (-109.6296, -4.9641)
  line L580 (-97.3491, -10.8536) -> (-97.3491, -9.3536)
  line L581 (-94.9444, -8.6036) -> (-96.2435, -9.3536)
  line L582 (-54.1852, -15.2432) -> (-55.4842, -15.9932)
  line L583 (-108.3306, -2.7141) -> (-109.6296, -1.9641)
  line L584 (-48.3519, -5.1395) -> (-49.6509, -5.8895)
  line L585 (-98.5185, -1.9641) -> (-99.8176, -2.7141)
  line L586 (-97.9472, -5.8895) -> (-97.9472, -7.3895)
  line L587 (-96.6481, -5.1395) -> (-97.9472, -5.8895)
  line L588 (-49.6509, -7.3895) -> (-48.3519, -8.1395)
  line L589 (-98.6481, -8.6036) -> (-99.9472, -9.3536)
  line L590 (-107.225, -4.2141) -> (-105.9259, -4.9641)
  line L591 (-70.6481, -5.1395) -> (-71.9472, -5.8895)
  line L592 (-62.1269, -20.6686) -> (-62.1269, -19.1686)
  line L593 (-108.9287, -0.75) -> (-107.6296, -1.5)
  line L594 (-55.4842, -15.9932) -> (-55.4842, -17.4932)
  line L595 (-49.5213, -0.75) -> (-48.2222, -1.5)
  line L596 (-65.701, -12.5291) -> (-67, -11.7791)
  line L597 (-97.8176, -0.75) -> (-96.5185, -1.5)
  line L598 (-107.7593, -5.1395) -> (-109.0583, -5.8895)
  line L599 (-55.8889, -11.7791) -> (-57.1879, -12.5291)
  line L600 (-107.6296, -1.5) -> (-106.3306, -0.75)
  line L601 (-97.9472, -7.3895) -> (-96.6481, -8.1395)
  line L602 (-59.1879, -17.4932) -> (-57.8889, -18.2432)
  line L603 (-107.225, -2.7141) -> (-107.225, -4.2141)
  line L604 (-71.9472, -7.3895) -> (-70.6481, -8.1395)
  line L605 (-72.1324, -20.6686) -> (-70.8333, -21.4186)
  line L606 (-92.9444, -5.1395) -> (-94.2435, -5.8895)
  line L607 (-63.2963, -11.7791) -> (-64.5953, -12.5291)
  line L608 (-109.6296, -4.9641) -> (-108.3306, -4.2141)
  line L609 (-71.8176, -0.75) -> (-70.5185, -1.5)
  line L610 (-52.7565, -9.3536) -> (-54.0556, -8.6036)
  line L611 (-100.9232, -2.7141) -> (-102.2222, -1.9641)
  line L612 (-72.5185, -1.9641) -> (-73.8176, -2.7141)
  line L613 (-91.6454, -5.8895) -> (-92.9444, -5.1395)
  line L614 (-94.8148, -4.9641) -> (-93.5158, -4.2141)
  line L615 (-75.0528, -9.3536) -> (-76.3519, -8.6036)
  line L616 (-102.2222, -1.9641) -> (-103.5213, -2.7141)
  line L617 (-102.4815, -18.2432) -> (-101.1824, -17.4932)
  line L618 (-100.0768, -15.9932) -> (-100.0768, -17.4932)
  line L619 (-97.4787, -17.4932) -> (-97.4787, -15.9932)
  line L620 (-101.7805, -14.0291) -> (-100.4815, -14.7791)
  line L621 (-98.0768, -14.0291) -> (-96.7778, -14.7791)
  line L622 (-103.7805, -17.4932) -> (-102.4815, -18.2432)
  line L623 (-102.4815, -15.2432) -> (-103.7805, -15.9932)
  line L624 (-99.1824, -14.0291) -> (-99.1824, -12.5291)
  line L625 (-96.299, -15.9932) -> (-96.299, -17.4932)
  line L626 (-110.1639, -5.8895) -> (-111.463, -5.1395)
  line L627 (-100.4815, -11.7791) -> (-101.7805, -12.5291)
  line L628 (-100.0768, -17.4932) -> (-98.7778, -18.2432)
  line L629 (-108.0185, -21.4186) -> (-106.7195, -20.6686)
  line L630 (-104.3148, -21.4186) -> (-103.0158, -20.6686)
  line L631 (-105.6139, -19.1686) -> (-105.6139, -20.6686)
  line L632 (-110.0343, 0.75) -> (-111.3333, 1.5)
  line L633 (-108.0185, -18.4186) -> (-109.3176, -19.1686)
  line L634 (-106.7195, -20.6686) -> (-106.7195, -19.1686)
  line L635 (-111.3333, -1.5) -> (-110.0343, -0.75)
  line L636 (-61.463, -8.6036) -> (-62.762, -9.3536)
  line L637 (-89.1667, -5.1395) -> (-90.4657, -5.8895)
  line L638 (-54.4602, -7.3895) -> (-54.4602, -5.8895)
  line L639 (-70.5185, -1.5) -> (-69.2195, -0.75)
  line L640 (-92.4101, -4.2141) -> (-91.1111, -4.9641)
  line L641 (-92.9444, -8.1395) -> (-91.6454, -7.3895)
  line L642 (-65.1667, -8.6036) -> (-66.4657, -9.3536)
  line L643 (-51.9259, -1.5) -> (-50.6269, -0.75)
  line L644 (-57.0583, -5.8895) -> (-57.0583, -7.3895)
  line L645 (-66.9444, -5.1395) -> (-68.2435, -5.8895)
  line L646 (-46.5185, -1.9641) -> (-47.8176, -2.7141)
  line L647 (-47.0528, -5.8895) -> (-48.3519, -5.1395)
  line L648 (-55.6296, -1.5) -> (-54.3306, -0.75)
  line L649 (-91.1667, -8.6036) -> (-92.4657, -9.3536)
  line L650 (-49.6509, -5.8895) -> (-49.6509, -7.3895)
  line L651 (-45.9472, -5.8895) -> (-45.9472, -7.3895)
  line L652 (-93.6454, -9.3536) -> (-94.9444, -8.6036)
  line L653 (-51.5213, -4.2141) -> (-50.2222, -4.9641)
  line L654 (-40.4101, -2.7141) -> (-40.4101, -4.2141)
  line L655 (-40.9444, -8.1395) -> (-39.6454, -7.3895)
  line L656 (-55.7593, -8.1395) -> (-54.4602, -7.3895)
  line L657 (-94.2435, -5.8895) -> (-94.2435, -7.3895)
  line L658 (-90.4657, -7.3895) -> (-89.1667, -8.1395)
  line L659 (-56.3306, -2.7141) -> (-57.6296, -1.9641)
  line L660 (-63.1667, -5.1395) -> (-64.4657, -5.8895)
  line L661 (-42.9444, -8.6036) -> (-44.2435, -9.3536)
  line L662 (-51.6509, -9.3536) -> (-51.6509, -10.8536)
  line L663 (-37.8121, -2.7141) -> (-39.1111, -1.9641)
  line L664 (-57.7593, -8.6036) -> (-59.0583, -9.3536)
  line L665 (-52.6269, -2.7141) -> (-53.9259, -1.9641)
  line L666 (-71.3491, -10.8536) -> (-71.3491, -9.3536)
  line L667 (-46.5185, -4.9641) -> (-45.2195, -4.2141)
  line L668 (-40.4101, -4.2141) -> (-39.1111, -4.9641)
  line L669 (-65.6454, -7.3895) -> (-65.6454, -5.8895)
  line L670 (-53.9259, -4.9641) -> (-52.6269, -4.2141)
  line L671 (-45.2195, -2.7141) -> (-46.5185, -1.9641)
  line L672 (-53.3546, -7.3895) -> (-52.0556, -8.1395)
  line L673 (-75.0528, -10.8536) -> (-75.0528, -9.3536)
  line L674 (-91.6454, -7.3895) -> (-91.6454, -5.8895)
  line L675 (-72.5185, -4.9641) -> (-71.2195, -4.2141)
  line L676 (-71.9472, -5.8895) -> (-71.9472, -7.3895)
  line L677 (-65.6454, -5.8895) -> (-66.9444, -5.1395)
  line L678 (-56.4602, -9.3536) -> (-57.7593, -8.6036)
  line L679 (-45.2195, -4.2141) -> (-45.2195, -2.7141)
  line L680 (-64.4101, -0.75) -> (-63.1111, -1.5)
  line L681 (-61.3333, -1.9641) -> (-62.6324, -2.7141)
  line L682 (-60.0343, -4.2141) -> (-60.0343, -2.7141)
  line L683 (-75.6509, -5.8895) -> (-75.6509, -7.3895)
  line L684 (-41.5158, -4.2141) -> (-41.5158, -2.7141)
  line L685 (-43.3491, -7.3895) -> (-43.3491, -5.8895)
  line L686 (-63.8676, -10.8536) -> (-63.8676, -9.3536)
  line L687 (-69.3491, -7.3895) -> (-69.3491, -5.8895)
  line L688 (-41.6454, -10.8536) -> (-41.6454, -9.3536)
  line L689 (-50.2222, -1.9641) -> (-51.5213, -2.7141)
  line L690 (-74.9232, -2.7141) -> (-76.2222, -1.9641)
  line L691 (-67.5158, -2.7141) -> (-68.8148, -1.9641)
  line L692 (-58.1639, -5.8895) -> (-59.463, -5.1395)
  line L693 (-72.6481, -8.6036) -> (-73.9472, -9.3536)
  line L694 (-62.6324, -4.2141) -> (-61.3333, -4.9641)
  line L695 (-47.8176, -2.7141) -> (-47.8176, -4.2141)
  line L696 (-93.6454, -10.8536) -> (-93.6454, -9.3536)
  line L697 (-45.9472, -7.3895) -> (-44.6481, -8.1395)
  line L698 (-58.9287, -2.7141) -> (-58.9287, -4.2141)
  line L699 (-37.1111, -1.5) -> (-35.8121, -0.75)
  line L700 (-44.6481, -5.1395) -> (-45.9472, -5.8895)
  line L701 (-61.8676, -7.3895) -> (-61.8676, -5.8895)
  line L702 (-44.6481, -8.1395) -> (-43.3491, -7.3895)
  line L703 (-59.0583, -9.3536) -> (-59.0583, -10.8536)
  line L704 (-48.2222, -1.5) -> (-46.9232, -0.75)
  line L705 (-39.6454, -5.8895) -> (-40.9444, -5.1395)
  line L706 (-38.4101, -0.75) -> (-37.1111, -1.5)
  line L707 (-68.2435, -7.3895) -> (-66.9444, -8.1395)
  line L708 (-60.1639, -10.8536) -> (-60.1639, -9.3536)
  line L709 (-50.2222, -4.9641) -> (-48.9232, -4.2141)
  line L710 (-55.225, -2.7141) -> (-55.225, -4.2141)
  line L711 (-89.8121, -2.7141) -> (-91.1111, -1.9641)
  line L712 (-92.4101, -2.7141) -> (-92.4101, -4.2141)
  line L713 (-66.8148, -1.5) -> (-65.5158, -0.75)
  line L714 (-68.8148, -1.9641) -> (-70.1139, -2.7141)
  line L715 (-60.762, -5.8895) -> (-60.762, -7.3895)
  line L716 (-63.1667, -8.1395) -> (-61.8676, -7.3895)
  line L717 (-45.3491, -9.3536) -> (-46.6481, -8.6036)
  line L718 (-66.4101, -4.2141) -> (-65.1111, -4.9641)
  line L719 (-67.5158, -4.2141) -> (-67.5158, -2.7141)
  line L720 (-43.3491, -5.8895) -> (-44.6481, -5.1395)
  line L721 (-45.8176, -0.75) -> (-44.5185, -1.5)
  line L722 (-39.1111, -1.9641) -> (-40.4101, -2.7141)
  line L723 (-40.8148, -1.5) -> (-39.5158, -0.75)
  line L724 (-50.3519, -8.6036) -> (-51.6509, -9.3536)
  line L725 (-55.3546, -9.3536) -> (-55.3546, -10.8536)
  line L726 (-50.7565, -5.8895) -> (-52.0556, -5.1395)
  line L727 (-60.1639, -9.3536) -> (-61.463, -8.6036)
  line L728 (-67.6454, -9.3536) -> (-68.9444, -8.6036)
  line L729 (-59.463, -8.1395) -> (-58.1639, -7.3895)
  line L730 (-52.7565, -10.8536) -> (-52.7565, -9.3536)
  line L731 (-49.0528, -10.8536) -> (-49.0528, -9.3536)
  line L732 (-60.0343, -2.7141) -> (-61.3333, -1.9641)
  line L733 (-56.3306, -4.2141) -> (-56.3306, -2.7141)
  line L734 (-64.4657, -7.3895) -> (-63.1667, -8.1395)
  line L735 (-89.8676, -9.3536) -> (-91.1667, -8.6036)
  line L736 (-57.6296, -4.9641) -> (-56.3306, -4.2141)
  line L737 (-52.6269, -4.2141) -> (-52.6269, -2.7141)
  line L738 (-62.6324, -2.7141) -> (-62.6324, -4.2141)
  line L739 (-67.6454, -10.8536) -> (-67.6454, -9.3536)
  line L740 (-39.6454, -7.3895) -> (-39.6454, -5.8895)
  line L741 (-61.8676, -5.8895) -> (-63.1667, -5.1395)
  line L742 (-44.5185, -1.5) -> (-43.2195, -0.75)
  line L743 (-64.4657, -5.8895) -> (-64.4657, -7.3895)
  line L744 (-47.0528, -7.3895) -> (-47.0528, -5.8895)
  line L745 (-51.5213, -2.7141) -> (-51.5213, -4.2141)
  line L746 (-42.2435, -5.8895) -> (-42.2435, -7.3895)
  line L747 (-55.7593, -5.1395) -> (-57.0583, -5.8895)
  line L748 (-48.9232, -4.2141) -> (-48.9232, -2.7141)
  line L749 (-57.0583, -7.3895) -> (-55.7593, -8.1395)
  line L750 (-70.2435, -9.3536) -> (-70.2435, -10.8536)
  line L751 (-48.9232, -2.7141) -> (-50.2222, -1.9641)
  line L752 (-53.225, -0.75) -> (-51.9259, -1.5)
  line L753 (-42.2435, -7.3895) -> (-40.9444, -8.1395)
  line L754 (-49.0528, -9.3536) -> (-50.3519, -8.6036)
  line L755 (-61.3333, -4.9641) -> (-60.0343, -4.2141)
  line L756 (-48.3519, -8.1395) -> (-47.0528, -7.3895)
  line L757 (-53.3546, -5.8895) -> (-53.3546, -7.3895)
  line L758 (-62.762, -9.3536) -> (-62.762, -10.8536)
  line L759 (-69.3491, -5.8895) -> (-70.6481, -5.1395)
  line L760 (-37.8121, -4.2141) -> (-37.8121, -2.7141)
  line L761 (-47.8176, -4.2141) -> (-46.5185, -4.9641)
  line L762 (-44.1139, -2.7141) -> (-44.1139, -4.2141)
  line L763 (-68.1139, -0.75) -> (-66.8148, -1.5)
  line L764 (-66.4101, -2.7141) -> (-66.4101, -4.2141)
  line L765 (-68.2435, -5.8895) -> (-68.2435, -7.3895)
  line L766 (-42.8148, -4.9641) -> (-41.5158, -4.2141)
  line L767 (-40.9444, -5.1395) -> (-42.2435, -5.8895)
  line L768 (-39.1111, -4.9641) -> (-37.8121, -4.2141)
  line L769 (-42.1139, -0.75) -> (-40.8148, -1.5)
  line L770 (-46.6481, -8.6036) -> (-47.9472, -9.3536)
  line L771 (-70.1139, -4.2141) -> (-68.8148, -4.9641)
  line L772 (-66.9444, -8.1395) -> (-65.6454, -7.3895)
  line L773 (-106.5899, -12.5291) -> (-107.8889, -11.7791)
  line L774 (-109.8889, -18.2432) -> (-108.5899, -17.4932)
  line L775 (-108.5899, -17.4932) -> (-108.5899, -15.9932)
  line L776 (-107.8889, -14.7791) -> (-106.5899, -14.0291)
  line L777 (-109.1879, -14.0291) -> (-107.8889, -14.7791)
  line L778 (-104.8861, -15.9932) -> (-106.1852, -15.2432)
  line L779 (-110.2936, -14.0291) -> (-110.2936, -12.5291)
  line L780 (-102.8861, -14.0291) -> (-102.8861, -12.5291)
  line L781 (-110.4232, -20.6686) -> (-110.4232, -19.1686)
  line L782 (-93.701, -15.9932) -> (-95, -15.2432)
  line L783 (-87.9973, -14.0291) -> (-87.9973, -12.5291)
  line L784 (-89.2963, -14.7791) -> (-87.9973, -14.0291)
  line L785 (-110.2936, -12.5291) -> (-111.5926, -11.7791)
  line L786 (-90.5953, -14.0291) -> (-89.2963, -14.7791)
  line L787 (-108.9287, 0.75) -> (-108.9287, -0.75)
  line L788 (-122.8333, -21.4186) -> (-121.5343, -20.6686)
  line L789 (-113.463, -8.6036) -> (-114.762, -9.3536)
  line L790 (-112.1639, -9.3536) -> (-113.463, -8.6036)
  line L791 (-121.5343, -19.1686) -> (-122.8333, -18.4186)
  line L792 (-46.9232, -0.75) -> (-46.9232, 0.75)
  line L793 (-56.9287, 0.75) -> (-56.9287, -0.75)
  line L794 (-113.3333, -1.9641) -> (-114.6324, -2.7141)
  line L795 (-122.8333, -18.4186) -> (-124.1324, -19.1686)
  line L796 (-68.1139, 0.75) -> (-68.1139, -0.75)
  line L797 (-116.4657, -5.8895) -> (-116.4657, -7.3895)
  line L798 (-58.0343, -0.75) -> (-58.0343, 0.75)
  line L799 (-112.762, -7.3895) -> (-111.463, -8.1395)
  line L800 (-112.0343, -2.7141) -> (-113.3333, -1.9641)
  line L801 (-115.8676, -9.3536) -> (-117.1667, -8.6036)
  line L802 (-49.5213, 0.75) -> (-49.5213, -0.75)
  line L803 (-60.6324, 0.75) -> (-60.6324, -0.75)
  line L804 (-112.6324, 0.75) -> (-112.6324, -0.75)
  line L805 (-72.9232, -0.75) -> (-72.9232, 0.75)
  line L806 (-83.3176, -19.1686) -> (-83.3176, -20.6686)
  line L807 (-114.6324, -2.7141) -> (-114.6324, -4.2141)
  line L808 (-115.1667, -8.1395) -> (-113.8676, -7.3895)
  line L809 (-124.1324, -19.1686) -> (-124.1324, -20.6686)
  line L810 (-113.5926, -15.2432) -> (-114.8916, -15.9932)
  line L811 (-114.8916, -15.9932) -> (-114.8916, -17.4932)
  line L812 (-111.463, -5.1395) -> (-112.762, -5.8895)
  line L813 (-119.701, -15.9932) -> (-121, -15.2432)
  line L814 (-79.225, 0.75) -> (-79.225, -0.75)
  line L815 (-121, -15.2432) -> (-122.299, -15.9932)
  line L816 (-117.1667, -8.6036) -> (-118.4657, -9.3536)
  line L817 (-112.2936, -15.9932) -> (-113.5926, -15.2432)
  line L818 (-112.0343, -4.2141) -> (-112.0343, -2.7141)
  line L819 (-112.762, -5.8895) -> (-112.762, -7.3895)
  line L820 (-116.725, -20.6686) -> (-115.4259, -21.4186)
  line L821 (-116.4657, -7.3895) -> (-115.1667, -8.1395)
  line L822 (-115.4259, -18.4186) -> (-116.725, -19.1686)
  line L823 (-85.7222, -21.4186) -> (-84.4232, -20.6686)
  line L824 (-87.8121, -0.75) -> (-87.8121, 0.75)
  line L825 (-124.1324, -20.6686) -> (-122.8333, -21.4186)
  line L826 (-115.9973, -15.9932) -> (-117.2963, -15.2432)
  line L827 (-115.2963, -11.7791) -> (-116.5953, -12.5291)
  line L828 (-77.0158, -20.6686) -> (-77.0158, -19.1686)
  line L829 (-112.2936, -17.4932) -> (-112.2936, -15.9932)
  line L830 (-98.9232, -0.75) -> (-98.9232, 0.75)
  line L831 (-114.6324, -4.2141) -> (-113.3333, -4.9641)
  line L832 (-102.6269, -0.75) -> (-102.6269, 0.75)
  line L833 (-87.0213, -19.1686) -> (-87.0213, -20.6686)
  line L834 (-113.8676, -7.3895) -> (-113.8676, -5.8895)
  line L835 (-82.0185, -18.4186) -> (-83.3176, -19.1686)
  line L836 (-115.1667, -5.1395) -> (-116.4657, -5.8895)
  line L837 (-116.5953, -14.0291) -> (-115.2963, -14.7791)
  line L838 (-114.8916, -17.4932) -> (-113.5926, -18.2432)
  line L839 (-76.6269, -0.75) -> (-76.6269, 0.75)
  line L840 (-117.2963, -15.2432) -> (-118.5953, -15.9932)
  line L841 (-38.4101, 0.75) -> (-38.4101, -0.75)
  line L842 (-113.8676, -5.8895) -> (-115.1667, -5.1395)
  line L843 (-113.3333, -4.9641) -> (-112.0343, -4.2141)
  line L844 (-35.8121, -0.75) -> (-35.8121, 0.75)
  line L845 (-39.5158, -0.75) -> (-39.5158, 0.75)
  line L846 (-113.5926, -18.2432) -> (-112.2936, -17.4932)
  line L847 (-113.0213, -20.6686) -> (-111.7222, -21.4186)
  line L848 (-110.0343, -0.75) -> (-110.0343, 0.75)
  line L849 (-45.8176, 0.75) -> (-45.8176, -0.75)
  line L850 (-115.2963, -14.7791) -> (-113.9973, -14.0291)
  line L851 (-116.5953, -12.5291) -> (-116.5953, -14.0291)
  line L852 (-118.4657, -10.8536) -> (-117.1667, -11.6036)
  line L853 (-112.8916, -12.5291) -> (-112.8916, -14.0291)
  line L854 (-113.463, -11.6036) -> (-112.1639, -10.8536)
  line L855 (-118.5953, -17.4932) -> (-117.2963, -18.2432)
  line L856 (-84.0343, -0.75) -> (-84.0343, 0.75)
  line L857 (-114.1269, -20.6686) -> (-114.1269, -19.1686)
  line L858 (-118.5953, -15.9932) -> (-118.5953, -17.4932)
  line L859 (-82.0185, -21.4186) -> (-80.7195, -20.6686)
  line L860 (-120.299, -14.0291) -> (-119, -14.7791)
  line L861 (-43.2195, -0.75) -> (-43.2195, 0.75)
  line L862 (-82.9287, 0.75) -> (-82.9287, -0.75)
  line L863 (-80.7195, -19.1686) -> (-82.0185, -18.4186)
  line L864 (-75.5213, 0.75) -> (-75.5213, -0.75)
  line L865 (-118.4657, -9.3536) -> (-118.4657, -10.8536)
  line L866 (-119, -14.7791) -> (-117.701, -14.0291)
  line L867 (-115.9973, -17.4932) -> (-115.9973, -15.9932)
  line L868 (-86.6324, 0.75) -> (-86.6324, -0.75)
  line L869 (-115.8676, -10.8536) -> (-115.8676, -9.3536)
  line L870 (-114.762, -10.8536) -> (-113.463, -11.6036)
  line L871 (-121, -18.2432) -> (-119.701, -17.4932)
  line L872 (-111.7222, -18.4186) -> (-113.0213, -19.1686)
  line L873 (-114.762, -9.3536) -> (-114.762, -10.8536)
  line L874 (-113.9973, -12.5291) -> (-115.2963, -11.7791)
  line L875 (-117.701, -12.5291) -> (-119, -11.7791)
  line L876 (-105.225, 0.75) -> (-105.225, -0.75)
  line L877 (-80.7195, -20.6686) -> (-80.7195, -19.1686)
  line L878 (-116.725, -19.1686) -> (-116.725, -20.6686)
  line L879 (-115.4259, -21.4186) -> (-114.1269, -20.6686)
  line L880 (-120.299, -12.5291) -> (-120.299, -14.0291)
  line L881 (-119, -11.7791) -> (-120.299, -12.5291)
  line L882 (-112.8916, -14.0291) -> (-111.5926, -14.7791)
  line L883 (-113.0213, -19.1686) -> (-113.0213, -20.6686)
  line L884 (-111.5926, -11.7791) -> (-112.8916, -12.5291)
  line L885 (-117.2963, -18.2432) -> (-115.9973, -17.4932)
  line L886 (-85.7222, -18.4186) -> (-87.0213, -19.1686)
  line L887 (-42.1139, 0.75) -> (-42.1139, -0.75)
  line L888 (-117.1667, -11.6036) -> (-115.8676, -10.8536)
  line L889 (-117.701, -14.0291) -> (-117.701, -12.5291)
  line L890 (-112.1639, -10.8536) -> (-112.1639, -9.3536)
  line L891 (-113.9973, -14.0291) -> (-113.9973, -12.5291)
  line L892 (-114.1269, -19.1686) -> (-115.4259, -18.4186)
  line L893 (-65.5158, -0.75) -> (-65.5158, 0.75)
  line L894 (-119.1296, -18.4186) -> (-120.4287, -19.1686)